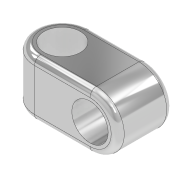
# Autodesk Inventor part: KNUCKLE_Dedao
Saved by Autodesk Inventor 2020 (Build 240168000, 168)
## iProperties
Created: 2021-04-01
Part Number: KNUCKLE_Dedao
Material: Generic
Document SubType Name: Modeling
Designer: deox
Density: 1 g/cm^3
Appearance: Chrome - Polished
Author: deox
Autodesk Inventor part; units mm, degrees
ref_plane "YZ Plane" through (0, 0, 0) normal (1, 0, 0) x (0, 1, 0)
ref_plane "XZ Plane" through (0, 0, 0) normal (0, 1, 0) x (-1, 0, 0)
ref_plane "XY Plane" through (0, 0, 0) normal (0, 0, 1) x (1, 0, 0)
sketch "Sketch1" plane through (0, 0, 0) normal (0, 0, 1) x (1, 0, 0)
  line L0 (-2.75, -1.375) -> (2.75, -1.375)
  line L1 (2.75, -1.375) -> (2.75, 1.375)
  line L2 (2.75, 1.375) -> (-2.75, 1.375)
  line L3 (-2.75, 1.375) -> (-2.75, -1.375)
  line L4 (-2.75, -1.375) -> (2.75, 1.375) construction
  line L5 (2.75, -1.375) -> (-2.75, 1.375) construction
  point P0 (0, 0)
  dimension "d0" = 5.5
  dimension "d1" = 2.75
  constraints: 12 end point, 2 midpoint, 2 parallel, 1 horizontal, 1 perpendicular
  measures "d0" distance of L2.end L1.end
  measures "d1" distance of L1.end L0.end
extrude "Extrusion1" add sketch "Sketch1" along normal mid plane 2.75
sketch "Sketch2" plane through (0, 0, 1.375) normal (0, 0, 1) x (1, 0, 0)
  circle A0 centre (1.375, 0) radius 1.375
  line L0 (2.75, 1.375) -> (-2.75, 1.375) projected
  line L1 (2.75, -1.375) -> (2.75, 1.375) projected
  line L2 (1.375, 0) -> (1.375, 1.375)
  line L3 (1.375, 1.375) -> (2.75, 1.375)
  line L4 (2.75, 1.375) -> (2.75, -1.375)
  line L5 (-2.75, -1.375) -> (2.75, -1.375) projected
  line L6 (2.75, -1.375) -> (1.375, -1.375)
  circle A1 centre (1.375, 0) radius 0.9
  point P0 (0, 0)
  point P1 (2.75, 0)
  dimension "d4" = 1.8
  constraints: 8 end point, 3 tangent, 2 centre point, 2 perpendicular, 2 point on circle, 2 point on line, 1 coincident
  measures "d4" diameter of A1
extrude "Extrusion2" cut sketch "Sketch2" against normal through all contours A1 | L1 L5 A0 | A0 L0 L1
sketch "Sketch3" plane through (-2.75, 1.375, 1.375) normal (0, 1, 0) x (1, 0, 0)
  line L0 (0, 2.75) -> (0, 0) projected
  line L1 (0, 1.375) -> (4.125, 1.375)
  line L2 (4.125, 2.75) -> (4.125, 0) projected
  circle A0 centre (1.375, 1.375) radius 1.375
  line L3 (0, 2.75) -> (4.125, 2.75) projected
  line L4 (0, 0) -> (0, 2.75) projected
  circle A1 centre (1.375, 1.375) radius 0.9
  line L5 (1.375, 1.375) -> (1.375, 0)
  line L6 (0, 0) -> (4.125, 0) projected
  line L7 (1.375, 0) -> (0, 0)
  line L8 (0, 0) -> (0, 2.75)
  line L9 (0, 2.75) -> (1.375, 2.75)
  point P0 (2.75, 1.375)
  dimension "d7" = 1.8
  constraints: 10 end point, 3 point on line, 2 centre point, 2 midpoint, 2 perpendicular, 2 point on circle, 2 tangent, 1 coincident
  measures "d7" diameter of A1
extrude "Extrusion3" cut sketch "Sketch3" against normal blind 2.75 contours L3 A0 L0 | A0 L6 L0 | A1 L1 | L1 L5 A1 | L1 A1 L5
fillet "Fillet1" radius 0.3248 8 edges at (0, 1.375, 1.375) (2.75, 0, 1.375) (0, -1.375, 1.375) (-2.75, -1.375, 0) (0, -1.375, -1.375) (2.75, 0, -1.375) (0, 1.375, -1.375) (-2.75, 1.375, 0)
body "Solid1"
